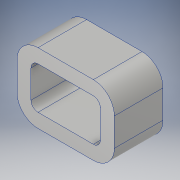
# Autodesk Inventor part: TestPoint_0603
Saved by Autodesk Inventor 2017 (Build 210142000, 142)
## iProperties
Created: 2017-07-25
Material: Zinc
Document SubType Name: Modeling
Designer: Bradley
Mass: 0.00539045 g
Surface Area: 0.0862137 cm^2
Volume: 0.000770064 cm^3
Density: 7 g/cm^3
Appearance: Aluminum - Flat
Description: RCU
Author: Bradley
Autodesk Inventor part; units mm, degrees
ref_plane "YZ Plane" through (0, 0, 0) normal (1, 0, 0) x (0, 1, 0)
ref_plane "XZ Plane" through (0, 0, 0) normal (0, 1, 0) x (-1, 0, 0)
ref_plane "XY Plane" through (0, 0, 0) normal (0, 0, 1) x (1, 0, 0)
sketch "Sketch1" plane through (0, 0, 0) normal (0, 0, 1) x (1, 0, 0)
  line L0 (-0.455, 0.575) -> (0.455, 0.575)
  line L1 (0.8, 0.23) -> (0.8, -0.23)
  line L2 (0.455, -0.575) -> (-0.455, -0.575)
  line L3 (-0.8, -0.23) -> (-0.8, 0.23)
  arc A0 (-0.455, 0.575) -> (-0.8, 0.23) centre (-0.455, 0.23) ccw
  arc A1 (0.8, 0.23) -> (0.455, 0.575) centre (0.455, 0.23) ccw
  arc A2 (0.455, -0.575) -> (0.8, -0.23) centre (0.455, -0.23) ccw
  arc A3 (-0.8, -0.23) -> (-0.455, -0.575) centre (-0.455, -0.23) ccw
  line L4 (-0.57, 0.23) -> (-0.57, -0.23)
  arc A4 (-0.57, -0.23) -> (-0.455, -0.345) centre (-0.455, -0.23) ccw
  line L5 (-0.455, -0.345) -> (0.455, -0.345)
  arc A5 (0.455, -0.345) -> (0.57, -0.23) centre (0.455, -0.23) ccw
  line L6 (0.57, -0.23) -> (0.57, 0.23)
  arc A6 (0.57, 0.23) -> (0.455, 0.345) centre (0.455, 0.23) ccw
  line L7 (0.455, 0.345) -> (-0.455, 0.345)
  arc A7 (-0.455, 0.345) -> (-0.57, 0.23) centre (-0.455, 0.23) ccw
  point P0 (0, 0)
  point P1 (-0.8, 0.575)
  point P2 (0.8, 0.575)
  point P3 (-0.8, -0.575)
  point P4 (0, 0.575)
  point P5 (-0.8, 0)
  dimension "d0" = 1.6
  dimension "d1" = 1.15
  dimension "d3" = 0.23
  dimension "d4" = 0.115
  constraints: 16 end point, 16 point on circle, 8 centre point, 8 tangent, 6 point on line, 4 parallel, 3 equal radius, 2 midpoint, 2 perpendicular, 1 horizontal, 1 horizontal alignment, 1 vertical alignment, 7 other
  measures "d0" distance of point (-0.8, 0.575) point (0.8, 0.575)
  measures "d1" distance of point (-0.8, -0.575) point (-0.8, 0.575)
  measures "d3" distance between parallel lines of L7 L0
  measures "d4" radius of A7
extrude "Extrusion1" add sketch "Sketch1" along normal mid plane 0.8
equation "\"d4\" = 0.5 * d3"
body "Solid1"
